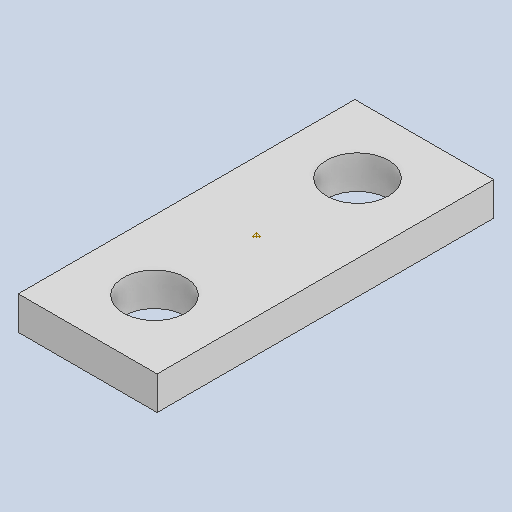
# Autodesk Inventor part: graphite_ledgereod
Saved by Autodesk Inventor 2024.2 (Build 282272000, 272)
## iProperties
Created: 2023-03-13
Part Number: graphite_ledgereod
Material: Generic
Document SubType Name: Modeling
Designer: warke
Density: 1 g/cm^3
Appearance: Default
Author: warke
Autodesk Inventor part; units mm, degrees
ref_plane "YZ Plane" through (0, 0, 0) normal (1, 0, 0) x (0, 1, 0)
ref_plane "XZ Plane" through (0, 0, 0) normal (0, 1, 0) x (-1, 0, 0)
ref_plane "XY Plane" through (0, 0, 0) normal (0, 0, 1) x (1, 0, 0)
sketch "Sketch2" plane through (0, 0, 0) normal (0, 1, 0) x (-1, 0, 0)
  line L0 (3.3, 8) -> (-3.3, 8)
  line L1 (-3.3, 8) -> (-3.3, -8)
  line L2 (-3.3, -8) -> (3.3, -8)
  line L3 (3.3, -8) -> (3.3, 8)
  line L4 (3.3, 8) -> (-3.3, -8) construction
  line L5 (-3.3, 8) -> (3.3, -8) construction
  point P0 (0, 0)
  dimension "d0" = 6.6
  dimension "d1" = 16
  constraints: 12 end point, 2 midpoint, 2 parallel, 1 horizontal, 1 perpendicular
  measures "d0" distance of L2.end L1.end
  measures "d1" distance of L1.end L0.end
extrude "Extrusion1" add sketch "Sketch2" along normal blind 1.5875
sketch "Sketch3" plane through (0, 1.5875, 0) normal (0, 1, 0) x (1, 0, 0)
  line L0 (-3.3, -8) -> (3.3, -8) projected
  line L1 (3.3, 8) -> (-3.3, 8) projected
  point P0 (0, 0)
  point P1 (0, 4.825)
  point P2 (0, -4.825)
hole "Hole1" at (0, 1.5875, -4.825) at (0, 1.5875, 4.825) direction (0, -1, 0) diameter 2.946 end through all clearance for "Flat Head Machine Screw (82)" size "#4" standard "Ansi Unified Screw Threads"
body "Solid1"
